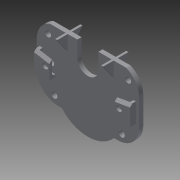
# Autodesk Inventor part: motor-holder
Saved by Autodesk Inventor 2014 (Build 180170000, 170)
## iProperties
Created: 2017-08-03
Part Number: motor-holder
Material: 一般
Document SubType Name: Modeling
Designer: hide
Density: 1 g/cm^3
Appearance: 既定
Author: hide
Autodesk Inventor part; units mm, degrees
ref_plane "YZ Plane" through (0, 0, 0) normal (1, 0, 0) x (0, 1, 0)
ref_plane "XZ Plane" through (0, 0, 0) normal (0, 1, 0) x (-1, 0, 0)
ref_plane "XY Plane" through (0, 0, 0) normal (0, 0, 1) x (1, 0, 0)
sketch "スケッチ8" plane through (0, 0, 0) normal (0, 1, 0) x (-1, 0, 0)
  line L0 (0, 0) -> (48.6, 0)
  line L1 (48.6, 0) -> (48.6, 32.6)
  line L2 (48.6, 32.6) -> (0, 32.6)
  line L3 (0, 32.6) -> (0, 0)
  circle A0 centre (5.3, 27.3) radius 1.5
  circle A1 centre (43.3, 27.3) radius 1.5
  circle A2 centre (8.3, 3.6) radius 1.5
  circle A3 centre (40.3, 3.6) radius 1.5
  circle A4 centre (24.3, 24.3) radius 5
  line L4 (19.3, 24.3) -> (29.3, 24.3)
  line L5 (29.3, 24.3) -> (29.3, 32.6)
  line L6 (29.3, 32.6) -> (19.3, 32.6)
  line L7 (19.3, 32.6) -> (19.3, 24.3)
  line L8 (0, 32.6) -> (48.6, 32.6)
  line L9 (48.6, 32.6) -> (48.6, 36.8)
  line L10 (48.6, 36.8) -> (0, 36.8)
  line L11 (0, 36.8) -> (0, 32.6)
  arc A5 (11.9042, 0) -> (36.6958, 0) centre (24.3, 10.7) ccw
  arc A6 (29.3, 25.8987) -> (29.0048, 25.9926) centre (24.3, 10.7) ccw
  arc A7 (19.5952, 25.9926) -> (19.3, 25.8987) centre (24.3, 10.7) ccw
  line L12 (11.9042, 0) -> (36.6958, 0)
  dimension "d42" = 32.6
  dimension "d43" = 48.6
  dimension "d44" = 3
  dimension "d45" = 3
  dimension "d46" = 3
  dimension "d47" = 3
  dimension "d48" = 38
  dimension "d49" = 32
  dimension "d50" = 5.3
  dimension "d51" = 8.3
  dimension "d52" = 5.3
  dimension "d53" = 0
  dimension "d54" = 3.6
  dimension "d55" = 0
  dimension "d56" = 10
  dimension "d57" = 19
  dimension "d58" = 8.3
  dimension "d61" = 36.8
  dimension "d103" = 10.7
  dimension "d104" = 0
  constraints: 26 end point, 9 point on circle, 8 centre point, 6 parallel, 6 point on line, 3 horizontal, 3 perpendicular, 1 collinear
  measures "d42" distance of L2.end L0.start
  measures "d43" distance of L0.start L0.end
  measures "d44" diameter of A0
  measures "d45" diameter of A1
  measures "d46" diameter of A2
  measures "d47" diameter of A3
  measures "d48" distance of A1.centre A0.centre
  measures "d49" distance of A3.centre A2.centre
  measures "d50" distance from line of L3 A0.centre
  measures "d51" distance from line of A2.centre L3
  measures "d52" distance from line of A0.centre L2
  measures "d53" vertical distance of A1.centre A0.centre
  measures "d54" distance from line of L0 A2.centre
  measures "d55" vertical distance of A3.centre A2.centre
  measures "d56" diameter of A4
  measures "d57" horizontal distance of A4.centre A0.centre
  measures "d58" distance from line of A4.centre L2
  measures "d61" distance between parallel lines of L0 L10
  measures "d103" distance from line of L0 A5.centre
  measures "d104" horizontal distance of A4.centre A5.centre
extrude "押し出し8" add sketch "スケッチ8" along normal blind 2 contours L3 L2 L7 A4 L5 L1 L0 | L0 A5
fillet "フィレット3" radius 10 4 edges at (0, 1, 32.6) (0, 1, 0) (-48.6, 1, 0) (-48.6, 1, 32.6)
sketch "スケッチ9" plane through (0, 0, 0) normal (0, -1, 0) x (1, 0, 0)
  line L0 (-10, 0) -> (-38.6, 0) projected
  line L1 (-48.5604, 35.5868) -> (6.5479, 35.5868)
  line L2 (6.5479, 35.5868) -> (6.5479, 31.8)
  line L3 (6.5479, 31.8) -> (-48.5604, 31.8)
  line L4 (-48.5604, 31.8) -> (-48.5604, 35.5868)
  point P0 (0, 0)
  dimension "d63" = 31.8
  constraints: 8 end point, 2 parallel, 1 horizontal, 1 perpendicular
  measures "d63" distance between parallel lines of L0 L3
extrude "押し出し9" cut sketch "スケッチ9" against normal blind 2
sketch "スケッチ10" plane through (0, 0, 0) normal (0, -1, 0) x (1, 0, 0)
  arc A0 (-29.3, 24.3) -> (-19.3, 24.3) centre (-24.3, 24.3) ccw projected
  line L0 (-47.1, 20.3) -> (-45.8, 20.3)
  line L1 (-45.8, 20.3) -> (-45.8, 11)
  line L2 (-45.8, 11) -> (-47.1, 11)
  line L3 (-47.1, 11) -> (-47.1, 20.3)
  line L4 (-47.1, 11) -> (-39.8, 11)
  line L5 (-39.8, 11) -> (-39.8, 12.3)
  line L6 (-39.8, 12.3) -> (-47.1, 12.3)
  line L7 (-47.1, 12.3) -> (-47.1, 11)
  line L8 (-1.5, 20.3) -> (-2.8, 20.3)
  line L9 (-2.8, 20.3) -> (-2.8, 11)
  line L10 (-2.8, 11) -> (-1.5, 11)
  line L11 (-1.5, 11) -> (-1.5, 20.3)
  line L12 (-1.5, 11) -> (-8.8, 11)
  line L13 (-8.8, 11) -> (-8.8, 12.3)
  line L14 (-8.8, 12.3) -> (-1.5, 12.3)
  line L15 (-1.5, 12.3) -> (-1.5, 11)
  point P0 (0, 0)
  dimension "d66" = 43
  dimension "d67" = 21.5
  dimension "d68" = 1.3
  dimension "d69" = 1.3
  dimension "d70" = 1.3
  dimension "d71" = 1.3
  dimension "d72" = 0
  dimension "d73" = 8
  dimension "d74" = 8
  dimension "d75" = 12
  dimension "d76" = 6
  dimension "d77" = 6
  constraints: 32 end point, 8 parallel, 4 horizontal, 4 perpendicular
  measures "d66" distance between parallel lines of L9 L1
  measures "d67" distance from line of A0.centre L1
  measures "d68" distance between parallel lines of L1 L3
  measures "d69" distance between parallel lines of L9 L11
  measures "d70" distance between parallel lines of L6 L4
  measures "d71" distance between parallel lines of L14 L12
  measures "d72" distance between parallel lines of L12 L4
  measures "d73" distance between parallel lines of L6 L0
  measures "d74" distance between parallel lines of L14 L8
  measures "d75" distance from line of A0.centre L6
  measures "d76" distance between parallel lines of L5 L1
  measures "d77" distance between parallel lines of L9 L13
extrude "押し出し10" add sketch "スケッチ10" along normal blind 1.5
sketch "スケッチ11" plane through (0, -1.5, 0) normal (0, -1, 0) x (1, 0, 0)
  line L0 (-45.8, 12.3) -> (-45.8, 20.3) projected
  line L1 (-45.8, 20.3) -> (-47.1, 20.3) projected
  line L2 (-47.1, 20.3) -> (-47.1, 11) projected
  line L3 (-47.1, 11) -> (-39.8, 11) projected
  line L4 (-39.8, 11) -> (-39.8, 12.3) projected
  line L5 (-39.8, 12.3) -> (-45.8, 12.3) projected
  line L6 (-47.1, 11) -> (-39.8, 11)
  line L7 (-39.8, 11) -> (-39.8, 20.3)
  line L8 (-39.8, 20.3) -> (-47.1, 20.3)
  line L9 (-47.1, 20.3) -> (-47.1, 11)
  line L10 (-1.5, 11) -> (-8.8, 11)
  line L11 (-8.8, 11) -> (-8.8, 20.3)
  line L12 (-8.8, 20.3) -> (-1.5, 20.3)
  line L13 (-1.5, 20.3) -> (-1.5, 11)
  point P0 (0, 0)
  constraints: 16 end point, 4 parallel, 2 horizontal, 2 perpendicular
extrude "押し出し11" add sketch "スケッチ11" along normal blind 1.3
sketch "スケッチ12" plane through (0, -2.8, 0) normal (0, -1, 0) x (1, 0, 0)
  line L0 (-47.1, 11) -> (-39.8, 11) projected
  line L1 (-39.8, 11) -> (-39.8, 20.3) projected
  line L2 (-39.8, 20.3) -> (-47.1, 20.3) projected
  line L3 (-47.1, 20.3) -> (-47.1, 11) projected
  circle A0 centre (-41.8, 16.3) radius 1.5
  circle A1 centre (-6.8, 16.3) radius 1.5
  arc A2 (-29.3, 24.3) -> (-19.3, 24.3) centre (-24.3, 24.3) ccw projected
  point P0 (0, 0)
  dimension "d82" = 3
  dimension "d83" = 3
  dimension "d84" = 35
  dimension "d85" = 17.5
  dimension "d86" = 0
  dimension "d87" = 8
  constraints: 2 centre point
  measures "d82" diameter of A0
  measures "d83" diameter of A1
  measures "d84" distance of A1.centre A0.centre
  measures "d85" horizontal distance of A2.centre A0.centre
  measures "d86" vertical distance of A1.centre A0.centre
  measures "d87" vertical distance of A0.centre A2.centre
extrude "押し出し12" cut sketch "スケッチ12" against normal blind 10 contours A0 | A1
chamfer "面取り3" distance 1.2 distance2 7 1 edges at (-39.8, -2.15, 20.3) measured on face at (-39.8, -2.3667, 14.5333)
chamfer "面取り4" distance 1.2 distance2 7 1 edges at (-8.8, -2.15, 20.3) measured on face at (-8.8, -2.3667, 14.5333)
chamfer "面取り5" distance 1.2 angle 45 2 edges at (-43.3, -2.8, 19.7) (-5.3, -2.8, 19.7)
sketch "スケッチ14" plane through (-19.3, 0, 31.8) normal (0, 0, 1) x (1, 0, 0)
  line L0 (13.2192, 0) -> (0, 0) projected
  line L1 (0, 2) -> (13.2192, 2) projected
  line L2 (-10, 2) -> (-10, 0) projected
  line L3 (-23.2192, 2) -> (-10, 2) projected
  line L4 (-23.2192, 0) -> (-23.2192, 2) projected
  line L5 (-10, 0) -> (-23.2192, 0) projected
  line L6 (-15.5703, 7) -> (-14.5703, 7)
  line L7 (-14.5703, 7) -> (-14.5703, -5)
  line L8 (-14.5703, -5) -> (-15.5703, -5)
  line L9 (-15.5703, -5) -> (-15.5703, 7)
  line L10 (6.2462, 7) -> (7.2462, 7)
  line L11 (7.2462, 7) -> (7.2462, -5)
  line L12 (7.2462, -5) -> (6.2462, -5)
  line L13 (6.2462, -5) -> (6.2462, 7)
  point P0 (19.3, 0)
  dimension "d114" = 1
  dimension "d115" = 1
  dimension "d116" = 5
  dimension "d117" = 5
  dimension "d118" = 5
  dimension "d119" = 5
  constraints: 16 end point, 4 parallel, 2 horizontal, 2 perpendicular
  measures "d114" distance of L6.start L6.end
  measures "d115" distance of L10.start L10.end
  measures "d116" distance between parallel lines of L3 L6
  measures "d117" distance between parallel lines of L1 L10
  measures "d118" distance between parallel lines of L0 L12
  measures "d119" distance between parallel lines of L5 L8
extrude "押し出し14" add sketch "スケッチ14" against normal blind 7 contours L11 L12 L13 L0 | L0 L13 L1 L11 | L1 L13 L10 L11 | L7 L5 L9 L3 | L3 L9 L6 L7 | L7 L8 L9 L5
chamfer "面取り6" distance 5 distance2 7 1 edges at (-12.5538, -5, 24.8) measured on face at (-12.7204, -1.6667, 24.8)
chamfer "面取り7" distance 5 distance2 7 1 edges at (-34.3703, -5, 24.8) measured on face at (-34.5369, -1.6667, 24.8)
chamfer "面取り8" distance 5 distance2 7 1 edges at (-12.5538, 7, 24.8) measured on face at (-12.7204, 5.3333, 24.8)
chamfer "面取り9" distance 5 distance2 7 1 edges at (-34.3703, 7, 24.8) measured on face at (-34.5369, 5.3333, 24.8)
fillet "フィレット5" radius 1 2 edges at (-42.8, -1.5, 12.3) (-5.8, -1.5, 12.3)
equation "\"d45\" = d44"
equation "\"d46\" = d44"
equation "\"d47\" = d44"
equation "\"d57\" = 0.5 * d48"
equation "\"d67\" = 0.5 * d66"
equation "\"d69\" = d68"
equation "\"d70\" = d68"
equation "\"d71\" = d70"
equation "\"d74\" = d73"
equation "\"d77\" = d76"
equation "\"d83\" = d82"
equation "\"d85\" = 0.5 * d84"
equation "\"d115\" = d114"
equation "\"d117\" = d116"
equation "\"d118\" = d117"
equation "\"d119\" = d116"
